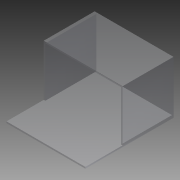
# Autodesk Inventor part: Bucket
Saved by Autodesk Inventor 2015 (Build 190159000, 159)
## iProperties
Created: 2015-03-01
Part Number: Bucket
Material: Polycarbonate, Clear
Document SubType Name: Modeling
Designer: patel_000
Density: 1.2 g/cm^3
Appearance: Polycarbonate - Clear
Author: patel_000
Autodesk Inventor part; units mm, degrees
ref_plane "YZ Plane" through (0, 0, 0) normal (1, 0, 0) x (0, 1, 0)
ref_plane "XZ Plane" through (0, 0, 0) normal (0, 1, 0) x (-1, 0, 0)
ref_plane "XY Plane" through (0, 0, 0) normal (0, 0, 1) x (1, 0, 0)
sketch "Sketch1" plane through (0, 0, 0) normal (0, 0, 1) x (1, 0, 0)
  line L0 (0, 0) -> (161.3408, 0)
  line L1 (161.3408, 0) -> (161.3408, 107.95)
  line L2 (161.3408, 107.95) -> (0, 107.95)
  line L3 (0, 107.95) -> (0, 0)
  line L4 (3.175, 3.175) -> (158.1658, 3.175)
  line L5 (158.1658, 3.175) -> (158.1658, 104.775)
  line L6 (158.1658, 104.775) -> (3.175, 104.775)
  line L7 (3.175, 104.775) -> (3.175, 3.175)
  dimension "d0" = 161.3408
  dimension "d1" = 107.95
  dimension "d2" = 154.9908
  dimension "d3" = 101.6
  dimension "d4" = 3.175
  dimension "d5" = 3.175
  constraints: 16 end point, 4 parallel, 2 horizontal, 2 perpendicular
  measures "d0" distance of L2.end L1.end
  measures "d1" distance of L1.end L0.end
  measures "d2" distance of L6.end L5.end
  measures "d3" distance of L5.end L4.end
  measures "d4" distance between parallel lines of L3 L7
  measures "d5" distance between parallel lines of L0 L4
extrude "Extrusion1" add sketch "Sketch1" against normal blind 180.34
sketch "Sketch2" plane through (161.3408, 0, 0) normal (1, 0, 0) x (0, 0, -1)
  line L0 (0, 3.175) -> (180.34, 3.175) projected
  line L1 (0, 107.95) -> (180.34, 107.95) projected
  line L2 (0, 3.175) -> (76.2, 3.175)
  line L3 (76.2, 3.175) -> (76.2, 107.95)
  line L4 (76.2, 107.95) -> (0, 107.95)
  line L5 (0, 107.95) -> (0, 3.175)
  point P0 (0, 0)
  dimension "d8" = 76.2
  constraints: 8 end point, 2 parallel, 1 horizontal, 1 perpendicular, 1 point on line
  measures "d8" distance of L4.end L3.end
extrude "Extrusion2" cut sketch "Sketch2" against normal through all
body "Solid1"
